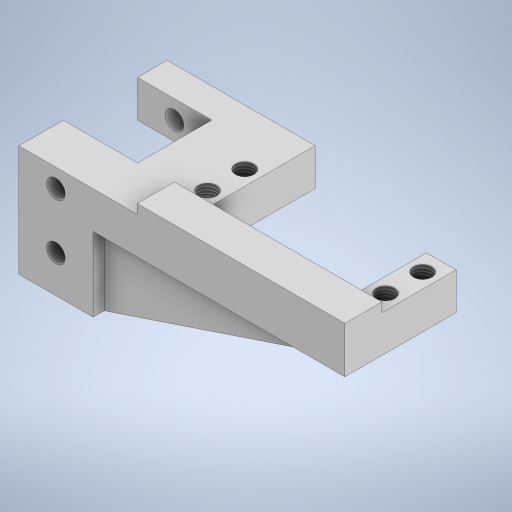
# Autodesk Inventor part: servo_holder
Saved by Autodesk Inventor 2024 (Build 280153000, 153)
## iProperties
Created: 2025-12-27
Part Number: servo_holder
Material: Generic
Document SubType Name: Modeling
Designer: schar
Density: 1 g/cm^3
Appearance: Default
Author: schar
Autodesk Inventor part; units mm, degrees
ref_plane "YZ Plane" through (0, 0, 0) normal (1, 0, 0) x (0, 1, 0)
ref_plane "XZ Plane" through (0, 0, 0) normal (0, 1, 0) x (-1, 0, 0)
ref_plane "XY Plane" through (0, 0, 0) normal (0, 0, 1) x (1, 0, 0)
ref_plane "Work Plane1" through (-26, 27.7, 10) normal (0, -1, 0) x (1, 0, 0)
sketch "Sketch1" plane through (-26, 27.7, 10) normal (0, -1, 0) x (1, 0, 0)
  line L0 (6, -0.5) -> (6, 0)
  line L1 (0, 0) -> (6.5, 0) projected
  line L2 (6, 0) -> (0, 0)
  line L3 (0, 0) -> (-2, 0)
  arc A0 (0, 0) -> (-2, -2) centre (0, -2) ccw projected
  line L4 (-2, 0) -> (-2, 0)
  line L5 (0, 0) -> (-2, 0)
  line L6 (-2, -2) -> (-2, -3.75) projected
  line L7 (-2, -2) -> (-2, 0)
  arc A1 (0, 0) -> (-2, -2) centre (0, -2) ccw projected
  line L8 (0, 0) -> (-2, 0)
  arc A2 (-2, -18) -> (0, -20) centre (0, -18) ccw projected
  line L9 (-2, -2) -> (-2, -18)
  line L10 (-2, -18) -> (-2, -20)
  line L11 (-2, -20) -> (0, -20)
  line L12 (0, -20) -> (6.5, -20)
  line L13 (6, -19.5) -> (6, -20)
  line L14 (6, -19.5) -> (6, -0.5)
  point P0 (26, -10)
  constraints: 26 end point, 7 tangent, 6 point on line, 4 vertical, 2 collinear, 2 perpendicular, 1 horizontal
extrude "Extrusion1" add sketch "Sketch1" along normal blind 10
ref_plane "Work Plane3" through (19.5, 27.7, -10) normal (0, -1, 0) x (1, 0, 0)
sketch "Sketch2" plane through (19.5, 27.7, -10) normal (0, -1, 0) x (1, 0, 0)
  line L0 (0.5, 19.5) -> (0.5, 0.5) projected
  line L1 (0.5, 19.5) -> (0.5, 20)
  line L2 (0, 20) -> (6.5, 20) projected
  line L3 (0.5, 0.4979) -> (0.5, -0.0021)
  arc A0 (6.5, 0) -> (8.5, 2) centre (6.5, 2) ccw projected
  line L4 (0, 0) -> (6.5, 0) projected
  line L5 (8.5, 2) -> (6.5, 2)
  line L6 (6.5, 2) -> (6.5, 0)
  line L7 (6.5, 0) -> (8.5, 0)
  line L8 (8.5, 0) -> (8.5, 2)
  line L9 (0.5, 20) -> (8.5, 20)
  line L10 (8.5, 20) -> (8.5, 0)
  line L11 (8.5, 0) -> (0.5, 0)
  line L12 (0.5, 0) -> (0.5, 20)
  point P0 (-19.5, 10)
  point P1 (0.5, 0.5)
  dimension "d4" = 0.5
  constraints: 20 end point, 4 parallel, 3 point on line, 2 horizontal, 2 perpendicular, 1 vertical
  measures "d4" distance of L3.start L3.end
extrude "Extrusion2" add sketch "Sketch2" along normal blind 10
ref_plane "Work Plane5" through (-19.5, 27.7, 10) normal (0, 0, 1) x (1, 0, 0)
sketch "Sketch3" plane through (-19.5, 27.7, 10) normal (0, 0, 1) x (1, 0, 0)
  line L0 (-8.5, 0) -> (-8.5, -10) projected
  line L1 (47.5, 0) -> (47.5, 2.5) projected
  line L2 (-8.5, -10) -> (47.5, -10)
  line L3 (47.5, -10) -> (47.5, 2.5)
  line L4 (47.5, 2.5) -> (-8.5, 2.5)
  line L5 (-8.5, 2.5) -> (-8.5, -10)
  point P0 (19.5, -27.7)
  constraints: 8 end point, 2 parallel, 1 horizontal, 1 perpendicular
extrude "Extrusion3" add sketch "Sketch3" along normal blind 10
ref_plane "Work Plane4" through (19.5, 27.7, -10) normal (0, 1, 0) x (1, 0, 0)
sketch "Sketch4" plane through (19.5, 27.7, -10) normal (0, 1, 0) x (1, 0, 0)
  arc A0 (6.415, -13.3929) -> (6.415, -16.6071) centre (4.5, -15) ccw projected
  circle A1 centre (4.5, -15) radius 2.5
  arc A2 (6.415, -3.3929) -> (6.415, -6.6071) centre (4.5, -5) ccw projected
  circle A3 centre (4.5, -5) radius 2.5
  arc A4 (-45.415, -16.6071) -> (-45.415, -13.3929) centre (-43.5, -15) ccw projected
  circle A5 centre (-43.5, -15) radius 2.5
  arc A6 (-45.415, -6.6071) -> (-45.415, -3.3929) centre (-43.5, -5) ccw projected
  circle A7 centre (-43.5, -5) radius 2.5
  point P0 (-19.5, -10)
  point P1 (6.415, -3.3929)
  point P2 (6.415, -13.3929)
  point P3 (-45.415, -16.6071)
  point P4 (-45.415, -6.6071)
  constraints: 4 coincident, 12 other
extrude "Extrusion4" cut sketch "Sketch4" against normal blind 10
ref_plane "Work Plane6" through (-28, 30.2, -3.75) normal (-1, 0, 0) x (0, 0, 1)
sketch "Sketch5" plane through (-28, 30.2, -3.75) normal (-1, 0, 0) x (0, 0, 1)
  line L0 (-6.25, -12.5) -> (23.75, -12.5) projected
  line L1 (-6.25, -2.5) -> (-6.25, -12.5) projected
  line L2 (23.75, -12.5) -> (-6.25, -12.5)
  line L3 (-6.25, -12.5) -> (-6.25, -2.5)
  line L4 (-6.25, -2.5) -> (23.75, -2.5)
  line L5 (23.75, -2.5) -> (23.75, -12.5)
  point P0 (3.75, -30.2)
  constraints: 8 end point, 2 parallel, 1 horizontal, 1 perpendicular
extrude "Extrusion5" add sketch "Sketch5" along normal blind 11.915
ref_plane "Work Plane7" through (19.5, 27.7, -10) normal (0, 0, -1) x (-1, 0, 0)
sketch "Sketch6" plane through (19.5, 27.7, -10) normal (0, 0, -1) x (-1, 0, 0)
  line L0 (39.5, 0) -> (39.5, -10) projected
  line L1 (47.5, 0) -> (59.415, 0) projected
  line L2 (39.5, -10) -> (59.415, -10)
  line L3 (59.415, -10) -> (59.415, 0)
  line L4 (59.415, 0) -> (39.5, 0)
  line L5 (39.5, 0) -> (39.5, -10)
  point P0 (19.5, -27.7)
  constraints: 8 end point, 2 parallel, 1 horizontal, 1 perpendicular
extrude "Extrusion6" add sketch "Sketch6" along normal blind 10
ref_plane "Work Plane8" through (-39.915, 30.2, -3.75) normal (-1, 0, 0) x (0, 0, 1)
sketch "Sketch7" plane through (-39.915, 30.2, -3.75) normal (-1, 0, 0) x (0, 0, 1)
  line L0 (-16.25, -12.5) -> (-16.25, -2.5) projected
  line L1 (-16.25, -12.5) -> (-6.25, -12.5)
  line L2 (-6.25, -12.5) -> (-6.25, -2.5)
  line L3 (-6.25, -2.5) -> (-16.25, -2.5)
  line L4 (-16.25, -2.5) -> (-16.25, -12.5)
  line L5 (23.75, -12.5) -> (23.75, -2.5) projected
  line L6 (23.75, -2.5) -> (13.75, -2.5)
  line L7 (13.75, -2.5) -> (13.75, -12.5)
  line L8 (13.75, -12.5) -> (23.75, -12.5)
  line L9 (23.75, -12.5) -> (23.75, -2.5)
  point P0 (3.75, -30.2)
  point P1 (23.75, -12.5)
  dimension "d15" = 10
  dimension "d16" = 10
  constraints: 16 end point, 4 parallel, 2 horizontal, 2 perpendicular, 1 point on line
  measures "d15" distance of L3.end L2.end
  measures "d16" distance of L8.end L7.end
extrude "Extrusion7" add sketch "Sketch7" along normal blind 20
ref_plane "Work Plane9" through (19.5, 27.7, -20) normal (0, 0, -1) x (-1, 0, 0)
sketch "Sketch9" plane through (-26, 17.7, 10) normal (0, -1, 0) x (1, 0, 0)
  line L0 (-13.915, 0) -> (-33.915, 0) projected
  line L1 (-13.915, 0) -> (-33.915, 0)
  line L2 (-33.915, 0) -> (-33.915, 10)
  line L3 (-33.915, 10) -> (-13.915, 10)
  line L4 (-13.915, 10) -> (-13.915, 0)
  point P0 (26, -10)
  point P1 (-33.915, 0)
  constraints: 8 end point, 2 parallel, 1 horizontal, 1 perpendicular
extrude "Extrusion9" add sketch "Sketch9" along normal blind 20
ref_plane "Work Plane2" through (-39.915, 27.7, 15) normal (0, 0, -1) x (-1, 0, 0)
sketch "Sketch10" plane through (-39.915, 27.7, 15) normal (0, 0, -1) x (-1, 0, 0)
  line L0 (20, -30) -> (0, -30) projected
  line L1 (-59.915, -10) -> (-67.915, -10) projected
  line L2 (0, -30) -> (-59.915, -10)
  line L3 (0, -30) -> (0, -10)
  line L4 (0, -10) -> (-59.915, -10)
  point P0 (-39.915, -27.7)
  constraints: 6 end point, 1 perpendicular
extrude "Extrusion10" add sketch "Sketch10" along normal mid plane 4
ref_plane "Work Plane10" through (-19.5, 27.7, 20) normal (0, 0, 1) x (1, 0, 0)
thread "Thread1" size "M5x0.8" class "6H" standard "ANSI Metric M Profile" length 15
thread "Thread2" size "M5x0.8" class "6H" standard "ANSI Metric M Profile" length 15
thread "Thread3" size "M5x0.8" class "6H" standard "ANSI Metric M Profile" length 15
thread "Thread4" size "M5x0.8" class "6H" standard "ANSI Metric M Profile" length 15
sketch "Sketch13" plane through (-19.5, 27.7, 20) normal (0, 0, 1) x (1, 0, 0)
  line L0 (-20.415, -10) -> (-20.415, 0) projected
  line L1 (-20.415, 0) -> (-30.415, 0)
  line L2 (-20.415, 0) -> (-40.415, 0) projected
  line L3 (-30.415, 0) -> (-30.415, -5)
  line L4 (-20.415, -10) -> (-20.415, -30) projected
  line L5 (-20.415, -30) -> (-20.415, -20)
  line L6 (-20.415, -20) -> (-30.415, -20)
  circle A0 centre (-30.415, -5) radius 2.5
  circle A1 centre (-30.415, -20) radius 2.5
  point P0 (19.5, -27.7)
  dimension "d40" = 10
  dimension "d41" = 5
  dimension "d42" = 10
  dimension "d43" = 10
  dimension "d44" = 5
  dimension "d45" = 5
  constraints: 8 end point, 2 centre point, 2 coincident, 2 midpoint, 1 perpendicular, 1 vertical
  measures "d40" distance of L0.end L1.end
  measures "d41" distance of L1.end L3.end
  measures "d42" distance of L4.end L5.end
  measures "d43" distance of L5.end L6.end
  measures "d44" diameter of A0
  measures "d45" diameter of A1
extrude "Extrusion12" cut sketch "Sketch13" against normal through all
sketch "Sketch14" plane through (-59.915, 27.7, -10) normal (0, 0, 1) x (1, 0, 0)
  line L0 (20, 0) -> (20, -10) projected
  line L1 (0, -10) -> (0, 0) projected
  line L2 (20, 0) -> (0, 0)
  line L3 (0, 0) -> (0, -10)
  line L4 (0, -10) -> (20, -10)
  line L5 (20, -10) -> (20, 0)
  point P0 (59.915, -27.7)
  point P1 (20, -10)
  constraints: 8 end point, 2 parallel, 1 horizontal, 1 perpendicular
extrude "Extrusion13" add sketch "Sketch14" against normal blind 2
sketch "Sketch15" plane through (-39.915, 27.7, 10) normal (0, 0, -1) x (-1, 0, 0)
  line L0 (20, -30) -> (0, -30) projected
  line L1 (20, 0) -> (0, 0)
  line L2 (0, 0) -> (0, -30)
  line L3 (0, -30) -> (20, -30)
  line L4 (20, -30) -> (20, 0)
  point P0 (-39.915, -27.7)
  constraints: 8 end point, 2 parallel, 1 horizontal, 1 perpendicular
extrude "Extrusion14" cut sketch "Sketch15" against normal blind 2
sketch "Sketch16" plane through (-39.915, 27.7, 12) normal (0, 0, -1) x (-1, 0, 0)
  line L0 (-11.915, 0) -> (20, 0) projected
  line L1 (20, -30) -> (0, -30) projected
  line L2 (20, 0) -> (0, 0)
  line L3 (0, 0) -> (0, -30)
  line L4 (0, -30) -> (20, -30)
  line L5 (20, -30) -> (20, 0)
  circle A0 centre (10, -20) radius 2.5 projected
  circle A1 centre (10, -20) radius 2.5
  circle A2 centre (10, -5) radius 2.5 projected
  circle A3 centre (10, -5) radius 2.5
  point P0 (-39.915, -27.7)
  point P1 (0, 0)
  constraints: 8 end point, 2 centre point, 2 coincident, 2 parallel, 1 horizontal, 1 perpendicular
extrude "Extrusion15" add sketch "Sketch16" along normal blind 4
sketch "Sketch17" plane through (-49.915, 22.7, -12) normal (0, 0, -1) x (-1, 0, 0)
  circle A0 centre (0, 0) radius 2.5
  point P0 (-49.915, -22.7)
  constraints: 1 centre point
extrude "Extrusion16" cut sketch "Sketch17" against normal blind 4
sketch "Sketch18" plane through (-59.915, 27.7, -10) normal (0, 0, 1) x (1, 0, 0)
  line L0 (0, -10) -> (0, 0) projected
  line L1 (20, 0) -> (0, 0) projected
  line L2 (0, -10) -> (20, -10)
  line L3 (20, -10) -> (20, 0)
  line L4 (20, 0) -> (0, 0)
  line L5 (0, 0) -> (0, -10)
  point P0 (59.915, -27.7)
  constraints: 8 end point, 2 parallel, 1 horizontal, 1 perpendicular
extrude "Extrusion17" cut sketch "Sketch18" against normal blind 2
body "Solid1"
body "Solid2"
